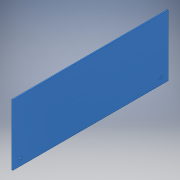
# Autodesk Inventor part: Side
Saved by Autodesk Inventor 2017 (Build 210142000, 142)
## iProperties
Created: 2017-11-22
Part Number: Side
Material: Generic
Document SubType Name: Modeling
Designer: guirguk
Density: 1 g/cm^3
Appearance: Cyan
Author: guirguk
Autodesk Inventor part; units mm, degrees
ref_plane "YZ Plane" through (0, 0, 0) normal (1, 0, 0) x (0, 1, 0)
ref_plane "XZ Plane" through (0, 0, 0) normal (0, 1, 0) x (-1, 0, 0)
ref_plane "XY Plane" through (0, 0, 0) normal (0, 0, 1) x (1, 0, 0)
sketch "Sketch1" plane through (0, 0, 0) normal (1, 0, 0) x (0, 1, 0)
  line L0 (0, 0) -> (200.025, 0)
  line L1 (200.025, 0) -> (200.025, -508)
  line L2 (200.025, -508) -> (0, -508)
  line L3 (0, -508) -> (0, 0)
  dimension "d0" = 200.025
  dimension "d1" = 508
  constraints: 8 end point, 3 perpendicular, 1 horizontal
  measures "d0" distance of L0.start L0.end
  measures "d1" distance of L0.end L1.end
extrude "Extrusion1" add sketch "Sketch1" along normal blind 3.175
sketch "Sketch3" plane through (3.175, 0, 0) normal (1, 0, 0) x (0, 0, -1)
  line L0 (0, 200.025) -> (0, 0) projected
  line L1 (0, 0) -> (0, 22.225)
  line L2 (0, 22.225) -> (25.4, 22.225)
  circle A0 centre (25.4, 22.225) radius 1.9844
  line L3 (0, 0) -> (508, 0) projected
  line L4 (508, 0) -> (508, 22.225)
  line L5 (508, 0) -> (508, 200.025) projected
  line L6 (508, 22.225) -> (482.6, 22.225)
  circle A1 centre (482.6, 22.225) radius 1.9844
  dimension "d8" = 22.225
  dimension "d9" = 25.4
  dimension "d10" = 3.9688
  dimension "d11" = 22.225
  dimension "d12" = 25.4
  dimension "d13" = 3.9688
  constraints: 8 end point, 2 centre point, 2 coincident, 2 perpendicular, 2 point on line
  measures "d8" distance of L0.end L1.end
  measures "d9" distance of L1.end L2.end
  measures "d10" diameter of A0
  measures "d11" distance of L3.end L4.end
  measures "d12" distance of L4.end L6.end
  measures "d13" diameter of A1
extrude "Extrusion2" cut sketch "Sketch3" against normal blind 3.175 contours A0
sketch "Sketch4" plane through (3.175, 0, 0) normal (1, 0, 0) x (0, 0, -1)
  line L0 (508, 0) -> (0, 0) projected
  line L1 (508, 0) -> (508, 22.225)
  line L2 (508, 200.025) -> (508, 0) projected
  line L3 (508, 22.225) -> (482.6, 22.225)
  circle A0 centre (482.6, 22.225) radius 1.9844
  dimension "d16" = 22.225
  dimension "d17" = 25.4
  dimension "d18" = 3.9688
  constraints: 4 end point, 1 centre point, 1 coincident, 1 perpendicular, 1 point on line
  measures "d16" distance of L0.start L1.end
  measures "d17" distance of L1.end L3.end
  measures "d18" diameter of A0
extrude "Extrusion3" cut sketch "Sketch4" against normal blind 3.175
sketch "Sketch5" plane through (3.175, 0, 0) normal (1, 0, 0) x (0, 0, -1)
  circle A0 centre (25.4, 22.225) radius 1.9844 projected
  circle A1 centre (25.4, 22.225) radius 3.9687
  point P0 (0, 0)
  dimension "d21" = 7.9375
  constraints: 1 centre point, 1 coincident
  measures "d21" diameter of A1
extrude "Extrusion4" cut sketch "Sketch5" against normal blind 3.175
sketch "Sketch6" plane through (3.175, 0, 0) normal (1, 0, 0) x (0, 0, -1)
  circle A0 centre (482.6, 22.225) radius 1.9844 projected
  circle A1 centre (482.6, 22.225) radius 3.9688
  point P0 (0, 0)
  dimension "d24" = 7.9375
  constraints: 1 centre point, 1 coincident
  measures "d24" diameter of A1
extrude "Extrusion5" cut sketch "Sketch6" against normal blind 3.175
body "Solid1"
